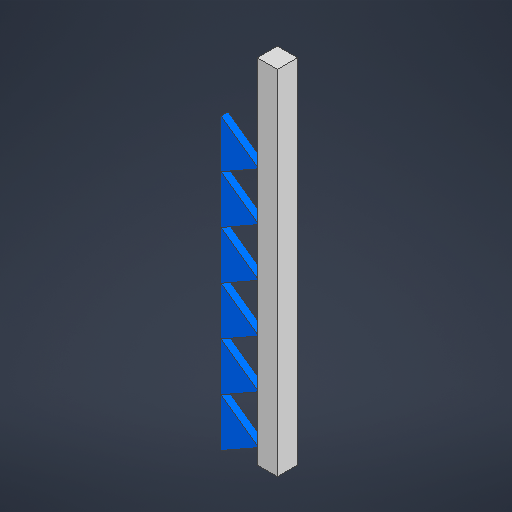
# Autodesk Inventor part: ДМФ 081 труба форсунки v2.0
Saved by Autodesk Inventor 2026.2 (Build 302298000, 298)
## iProperties
Created: 2024-06-28
Part Number: ДМФ 081 труба форсунки v2.0
Material: Generic
Document SubType Name: Modeling
Designer: admin
Density: 1 g/cm^3
Appearance: Default
Author: admin
Autodesk Inventor part; units mm, degrees
ref_plane "YZ Plane" through (0, 0, 0) normal (1, 0, 0) x (0, 1, 0)
ref_plane "XZ Plane" through (0, 0, 0) normal (0, 1, 0) x (-1, 0, 0)
ref_plane "XY Plane" through (0, 0, 0) normal (0, 0, 1) x (1, 0, 0)
sketch "Sketch2" plane through (0, 0, 0) normal (0, 0, 1) x (1, 0, 0)
  line L0 (-20, 20) -> (20, 20)
  line L1 (20, 20) -> (20, -20)
  line L2 (20, -20) -> (-20, -20)
  line L3 (-20, -20) -> (-20, 20)
  line L4 (-20, 20) -> (20, -20) construction
  line L5 (20, 20) -> (-20, -20) construction
  point P0 (0, 0)
  dimension "d8" = 40
  dimension "d9" = 40
  constraints: 12 end point, 2 midpoint, 2 parallel, 1 horizontal, 1 perpendicular
  measures "d8" distance of L1.end L2.end
  measures "d9" distance of L0.end L1.end
extrude "Extrusion2" add sketch "Sketch2" against normal blind 700
sketch "Sketch3" plane through (0, 0, 0) normal (0, 1, 0) x (-1, 0, 0)
  line L0 (20, 0) -> (-20, 0) construction
  line L1 (20, 0) -> (20, -700) construction
  line L2 (-20, -700) -> (20, -700) construction
  line L3 (-20, 0) -> (-20, -700) construction
  line L4 (0, -673) -> (30, -673)
  line L5 (30, -673) -> (30, -690)
  line L6 (30, -690) -> (0, -690)
  line L7 (0, -690) -> (0, -673)
  line L8 (0, -673) -> (30, -690) construction
  line L9 (30, -673) -> (0, -690) construction
  line L10 (30, -681.5) -> (104.9319, -628.1281)
  line L11 (104.9319, -628.1281) -> (104.9319, -723.9614)
  line L12 (104.9319, -723.9614) -> (30, -681.5)
  point P0 (0, 0)
  point P1 (15, -681.5)
  dimension "d10" = 30
  dimension "d11" = 17
  dimension "d12" = 65
  dimension "d13" = 10
  dimension "d14" = 20
  dimension "d15" = 95.8333
  constraints: 18 end point, 3 midpoint, 3 parallel, 1 horizontal, 1 perpendicular, 1 vertical
  measures "d10" distance of L5.end L6.end
  measures "d11" distance of L4.end L5.end
  measures "d12" angle of L12 L10
  measures "d13" distance between parallel lines of L2 L6
  measures "d14" distance between parallel lines of L3 L7
  measures "d15" distance of L10.end L11.end
extrude "Extrusion3" add sketch "Sketch3" along normal mid plane 14
pattern_linear "Rectangular Pattern1" count 6 spacing 95.8333 along (0, 0, 1) of "Extrusion3"
equation "\"d15\" = ширина_факела"
equation "\"d20\" = ширина_факела"
equation "\"ширина_факела\" = 95.83333"
body "Solid2"
